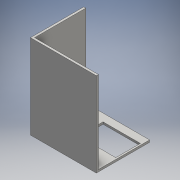
# Autodesk Inventor part: RoomEnvironment
Saved by Autodesk Inventor 2016 (Build 200138000, 138)
## iProperties
Created: 2015-11-22
Part Number: RoomEnvironment
Material: 常规
Document SubType Name: Modeling
Designer: Shawn Shi Feng
Density: 1 g/cm^3
Appearance: 默认
Author: Shawn Shi Feng
Autodesk Inventor part; units mm, degrees
ref_plane "YZ Plane" through (0, 0, 0) normal (1, 0, 0) x (0, 1, 0)
ref_plane "XZ Plane" through (0, 0, 0) normal (0, 1, 0) x (-1, 0, 0)
ref_plane "XY Plane" through (0, 0, 0) normal (0, 0, 1) x (1, 0, 0)
sketch "草图1" plane through (0, 0, 0) normal (0, 0, 1) x (1, 0, 0)
  line L0 (-155.9868, 158.5636) -> (156.5132, 158.5636)
  line L1 (156.5132, 158.5636) -> (156.5132, -93.9364)
  line L2 (156.5132, -93.9364) -> (-155.9868, -93.9364)
  line L3 (-155.9868, -93.9364) -> (-155.9868, 158.5636)
  line L4 (-27.9868, 122.5636) -> (149.0132, 122.5636)
  line L5 (149.0132, 122.5636) -> (149.0132, 5.5636)
  line L6 (149.0132, 5.5636) -> (-27.9868, 5.5636)
  line L7 (-27.9868, 5.5636) -> (-27.9868, 122.5636)
  line L8 (-155.9868, -83.9364) -> (-155.9868, 158.5636)
  line L9 (-155.9868, -93.9364) -> (156.5132, -93.9364)
  line L10 (156.5132, -93.9364) -> (156.5132, -83.9364)
  line L11 (-155.9868, -83.9364) -> (-155.9868, -93.9364)
  point P0 (0, 0)
  dimension "d0" = 312.5
  dimension "d1" = 252.5
  dimension "d2" = 36
  dimension "d3" = 7.5
  dimension "d4" = 177
  dimension "d5" = 117
  constraints: 24 end point, 5 parallel, 3 horizontal, 3 perpendicular, 1 point on line
  measures "d0" distance of L1.end L2.end
  measures "d1" distance of L0.end L1.end
  measures "d2" distance between parallel lines of L4 L0
  measures "d3" distance between parallel lines of L1 L5
  measures "d4" distance of L5.end L6.end
  measures "d5" distance of L4.end L5.end
extrude "拉伸1" add sketch "草图1" against normal blind 10
sketch "草图3" plane through (0, 0, 0) normal (0, 0, 1) x (1, 0, 0)
  line L0 (-155.9868, 158.5636) -> (156.5132, 158.5636) projected
  line L1 (-145.9868, 158.5636) -> (-155.9868, 158.5636)
  line L2 (-155.9868, 158.5636) -> (-155.9868, -93.9364)
  line L3 (-155.9868, -93.9364) -> (-145.9868, -93.9364)
  line L4 (-145.9868, -93.9364) -> (-145.9868, 158.5636)
  point P0 (0, 0)
  dimension "d16" = 10
  constraints: 8 end point, 2 parallel, 1 horizontal, 1 perpendicular, 1 point on line
  measures "d16" distance between parallel lines of L4 L2
extrude "拉伸2" add sketch "草图3" along normal blind 390
sketch "草图4" plane through (0, 0, 0) normal (0, 0, 1) x (1, 0, 0)
  line L0 (156.5132, -93.9364) -> (-145.9868, -93.9364) projected
  line L1 (-145.9868, 148.5636) -> (-145.9868, -93.9364) projected
  line L2 (156.5132, -93.9364) -> (-145.9868, -93.9364)
  line L3 (-145.9868, -93.9364) -> (-145.9868, -83.9364)
  line L4 (-145.9868, -83.9364) -> (156.5132, -83.9364)
  line L5 (156.5132, -83.9364) -> (156.5132, -93.9364)
  point P0 (0, 0)
  dimension "d13" = 10
  constraints: 8 end point, 2 parallel, 1 horizontal, 1 perpendicular, 1 point on line
  measures "d13" distance between parallel lines of L0 L4
extrude "拉伸3" add sketch "草图4" along normal blind 390
